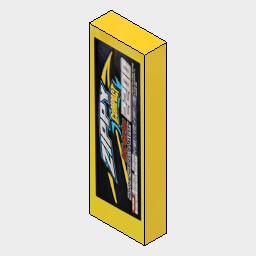
Battery (Autodesk Fusion 360 design; units mm, degrees)
Autodesk Fusion 360 part; units mm, degrees
sketch "Sketch1" plane through (0, 0, 0) normal (0, 1, 0) x (1, 0, 0)
  line L0 (0, 0) -> (35, 0)
  line L1 (35, 0) -> (35, -14)
  line L2 (0, -14) -> (0, 0)
  line L3 (0, 0) -> (35, 0)
  line L4 (35, 0) -> (35, -14)
  line L5 (35, -14) -> (0, -14)
  line L6 (0, -14) -> (0, 0)
  dimension "d6" = 35
  dimension "d8" = 14
  measures "d6" distance of L0.start L0.end
  measures "d8" distance of L0.start L2.start
extrude "Extrude1" add sketch "Sketch1" along normal blind 104
